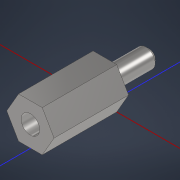
# Autodesk Inventor part: M3x10x6 Standoff
Saved by Autodesk Inventor 2022.2 (Build 262287010, 287A)
## iProperties
Created: 2022-03-13
Part Number: M3x10x6 Standoff
Material: Edelstahl
Document SubType Name: Modeling
Designer: sleib
Density: 8 g/cm^3
Appearance: Halbpoliert
Author: sleib
Autodesk Inventor part; units mm, degrees
ref_plane "YZ Plane" through (0, 0, 0) normal (1, 0, 0) x (0, 1, 0)
ref_plane "XZ Plane" through (0, 0, 0) normal (0, 1, 0) x (-1, 0, 0)
ref_plane "XY Plane" through (0, 0, 0) normal (0, 0, 1) x (1, 0, 0)
sketch "Skizze1" plane through (0, 0, 0) normal (0, 0, 1) x (1, 0, 0)
  line L0 (1.5877, 2.75) -> (3.1754, 0)
  line L1 (3.1754, 0) -> (1.5877, -2.75)
  line L2 (1.5877, -2.75) -> (-1.5877, -2.75)
  line L3 (-1.5877, -2.75) -> (-3.1754, 0)
  line L4 (-3.1754, 0) -> (-1.5877, 2.75)
  line L5 (-1.5877, 2.75) -> (1.5877, 2.75)
  circle A0 centre (0, 0) radius 1.25
  circle A1 centre (0, 0) radius 1.5
  point P0 (0, -2.75)
  dimension "d0" = 5.5
  dimension "d1" = 2.5
  dimension "d2" = 3
  constraints: 12 end point, 3 coincident, 2 centre point, 1 horizontal, 1 midpoint, 13 other
  measures "d0" distance from line of point (0, -2.75) L5
  measures "d1" diameter of A0
  measures "d2" diameter of A1
extrude "Extrusion1" add sketch "Skizze1" along normal blind 10 contours L0 L1 L2 L3 L4 L5 | A1
extrude "Extrusion2" add sketch "Skizze1" along normal blind 2 contours A0
extrude "Extrusion3" add sketch "Skizze1" against normal blind 6 contours A0
chamfer "Fase1" distance 0.5 angle 45 1 edges at (-1.25, 0, -6)
